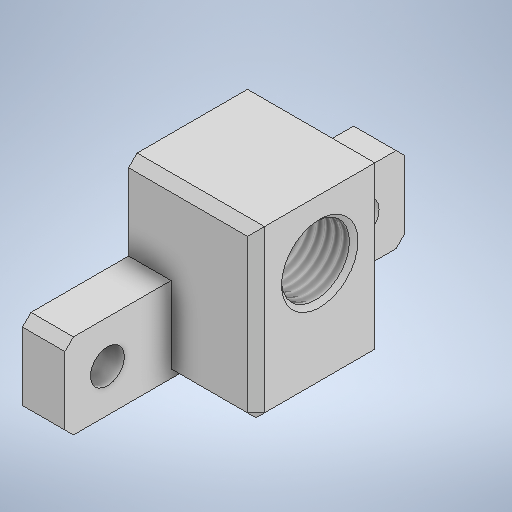
# Autodesk Inventor part: chain piston adaptor
Saved by Autodesk Inventor 2026.1 (Build 301233020, 233B)
## iProperties
Created: 2026-01-23
Part Number: chain piston adaptor
Material: Generic
Document SubType Name: Modeling
Designer: user
Density: 1 g/cm^3
Appearance: Default
Author: user
Autodesk Inventor part; units mm, degrees
ref_plane "YZ Plane" through (0, 0, 0) normal (1, 0, 0) x (0, 1, 0)
ref_plane "XZ Plane" through (0, 0, 0) normal (0, 1, 0) x (-1, 0, 0)
ref_plane "XY Plane" through (0, 0, 0) normal (0, 0, 1) x (1, 0, 0)
sketch "Sketch1" plane through (0, 0, 0) normal (1, 0, 0) x (0, 1, 0)
  line L0 (-5, 20) -> (5, 20)
  line L1 (5, 20) -> (5, -20)
  line L2 (5, -20) -> (-5, -20)
  line L3 (-5, -20) -> (-5, 20)
  line L4 (-5, 20) -> (5, -20) construction
  line L5 (5, 20) -> (-5, -20) construction
  line L6 (-7.5, 7.5) -> (7.5, -7.5) construction
  line L7 (7.5, 7.5) -> (-7.5, -7.5) construction
  line L8 (15, -7.5) -> (15, 7.5)
  line L9 (15, 7.5) -> (-5, 7.5)
  line L10 (-15, -7.5) -> (15, 7.5) construction
  line L11 (15, -7.5) -> (-15, 7.5) construction
  line L12 (-5, -7.5) -> (15, -7.5)
  point P0 (0, 0)
  point P1 (5, -7.5)
  point P2 (5, 7.5)
  point P3 (5, -7.5)
  dimension "d0" = 10
  dimension "d1" = 40
  dimension "d3" = 15
  dimension "d32" = 10
  dimension "d33" = 40
  constraints: 26 end point, 7 midpoint, 3 parallel, 2 horizontal, 2 perpendicular, 2 point on line
  measures "d0" distance of L1.end L2.end
  measures "d1" distance of L0.end L1.end
  measures "d3" distance of L7.start L6.end
  measures "d32" distance of point (5, -7.5) L8.start
  measures "d33" distance of L2.end L0.start
extrude "Extrusion1" add sketch "Sketch1" along normal blind 5
sketch "Sketch4" plane through (0, 0, 0) normal (-1, 0, 0) x (0, 0, 1)
  line L0 (-20, -5) -> (-20, 5) projected
  line L1 (-20, 0) -> (-17, 0)
  line L2 (-17, 0) -> (-15, 0)
  circle A0 centre (-15, 0) radius 2
  line L3 (20, 5) -> (20, -5) projected
  circle A1 centre (15, 0) radius 2
  point P0 (0, 0)
  point P1 (-20, -4)
  point P2 (-20, 4)
  point P3 (20, 4)
  point P4 (20, -4)
  dimension "d25" = 3
  dimension "d26" = 2
  dimension "d28" = 4
  constraints: 4 end point, 1 centre point, 1 coincident, 1 horizontal, 1 horizontal alignment, 1 midpoint, 1 point on line, 2 other
  measures "d25" distance of L1.start L1.end
  measures "d26" distance of L1.end L2.end
  measures "d28" diameter of A1
extrude "Extrusion4" cut sketch "Sketch4" against normal blind 10
sketch "Sketch5" plane through (5, 0, 0) normal (1, 0, 0) x (0, 0, -1)
  line L0 (7.5, 15) -> (-7.5, 15) projected
  line L1 (-7.5, 15) -> (-7.5, -5)
  line L2 (-20, -5) -> (20, -5) projected
  line L3 (-7.5, 15) -> (7.5, 15)
  line L4 (7.5, 5) -> (7.5, 15) projected
  line L5 (7.5, 5) -> (7.5, 15)
  line L6 (7.5, 15) -> (7.5, 5)
  line L7 (7.5, -5) -> (-7.5, -5)
  line L8 (7.5, 5) -> (7.5, -5)
  line L9 (-7.5, -5) -> (7.5, -5)
  point P0 (0, 0)
  constraints: 14 end point, 4 collinear, 2 perpendicular, 2 point on line, 1 vertical
extrude "Extrusion5" add sketch "Sketch5" along normal blind 10
sketch "Sketch6" plane through (15, 0, 0) normal (1, 0, 0) x (0, 0, -1)
  line L0 (7.5, 15) -> (-7.5, 15) projected
  circle A0 centre (0, 8) radius 4
  point P0 (0, 0)
  point P1 (0, 15)
  dimension "d37" = 8
  dimension "d40" = 7
  constraints: 1 centre point, 1 midpoint
  measures "d37" diameter of A0
  measures "d40" distance of point (0, 15) A0.centre
extrude "Extrusion6" cut sketch "Sketch6" against normal blind 10
thread "Thread2" size "M8x1" class "6H" standard "ANSI Metric M Profile" length 20
chamfer "Chamfer5" distance 1 angle 45 11 edges at (7.5, 15, 7.5) (7.5, 15, -7.5) (15, 5, -7.5) (15, 5, 7.5) (15, -5, 0) (10, -5, 7.5) (2.5, 5, 20) (2.5, -5, 20) (2.5, 5, -20) (2.5, -5, -20) (10, -5, -7.5)
chamfer "Chamfer6" distance 0.5 angle 45 1 edges at (15, 8, 4)
body "Solid1"
